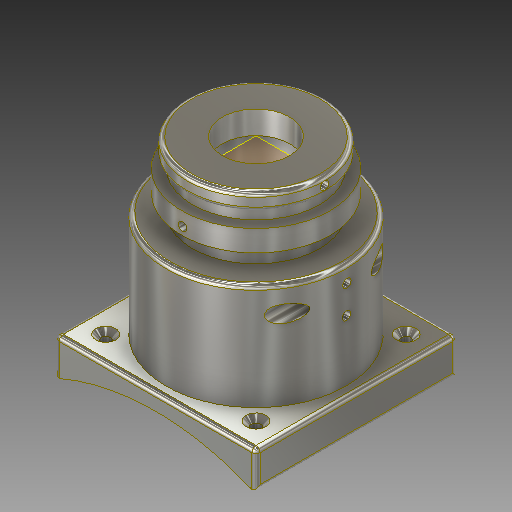
# Autodesk Inventor part: wyciag
Saved by Autodesk Inventor 2019.4 (Build 234330000, 330)
## iProperties
Created: 2019-06-01
Part Number: wyciag
Material: Silver
Document SubType Name: Modeling
Designer: Esterka
Density: 10.49 g/cm^3
Appearance: Silver
Author: Esterka
Autodesk Inventor part; units mm, degrees
ref_plane "XZ Plane" through (0, 0, 0) normal (0, 1, 0) x (-1, 0, 0)
sketch "Sketch1" plane through (0, 0, 0) normal (0, 0, 1) x (1, 0, 0)
  line L0 (0, 0) -> (95, 0)
  line L1 (0, 0) -> (0, -18)
  line L2 (95, -18) -> (95, 0)
  arc A0 (95, -18) -> (0, -18) centre (47.5, -122.7318) ccw
  dimension "d0" = 95
  dimension "d22" = 18
  dimension "d23" = 230
  dimension "d83" = 90
  dimension "d84" = 47.5
  constraints: 6 end point, 2 point on circle, 1 centre point, 1 horizontal, 1 vertical
  measures "d0" distance of L0.start L0.end
  measures "d22" distance of L0.start L1.end
  measures "d23" diameter of A0
  measures "d83" angle of L0 L2
  measures "d84" horizontal distance of L0.end A0.centre
extrude "Extrusion1" add sketch "Sketch1" along normal blind 95
fillet "Fillet1" radius 2 4 edges at (47.5, 0, 0) (0, 0, 47.5) (47.5, 0, 95) (95, 0, 47.5)
sketch "Sketch2" plane through (2, 0, 2) normal (0, 1, 0) x (1, 0, 0)
  line L0 (-1, 0) -> (-1, -98) projected
  circle A0 centre (45.5, -45.5) radius 42.5
  line L1 (93, 2) -> (-2, 2) projected
  line L2 (-2, 2) -> (-2, -93) projected
  dimension "d7" = 85
  dimension "d26" = 47.5
  dimension "d27" = 47.5
  constraints: 1 centre point, 1 coincident
  measures "d7" diameter of A0
  measures "d26" distance from line of L1 point (45.5, -45.5)
  measures "d27" distance from line of L2 point (45.5, -45.5)
extrude "Extrusion2" add sketch "Sketch2" along normal blind 50
sketch "Sketch3" plane through (47.5, 50, 47.5) normal (0, 1, 0) x (1, 0, 0)
  circle A0 centre (0, 0) radius 30
  point P0 (-47.5, 47.5)
  dimension "d10" = 60
  constraints: 1 centre point
  measures "d10" diameter of A0
extrude "Extrusion3" add sketch "Sketch3" along normal blind 23
fillet "Fillet2" radius 2 1 edges at (5, 50, 47.5)
ref_plane "Work Plane1" through (47.5, 68, 47.5) normal (0, 1, 0) x (1, 0, 0)
sketch "Sketch4" plane through (47.5, 68, 47.5) normal (0, 1, 0) x (1, 0, 0)
  circle A0 centre (0, 0) radius 35
  point P0 (-47.5, 47.5)
  dimension "d15" = 70
  constraints: 1 centre point
  measures "d15" diameter of A0
extrude "Extrusion4" add sketch "Sketch4" against normal blind 10
sketch "Sketch5" plane through (47.5, 73, 47.5) normal (0, 1, 0) x (1, 0, 0)
  circle A0 centre (0, 0) radius 32.5
  point P0 (-47.5, 47.5)
  dimension "d18" = 65
  constraints: 1 centre point
  measures "d18" diameter of A0
extrude "Extrusion5" add sketch "Sketch5" along normal blind 8
sketch "Sketch6" plane through (47.5, 81, 47.5) normal (0, 1, 0) x (1, 0, 0)
  circle A0 centre (0, 0) radius 15.875
  point P0 (-47.5, 47.5)
  dimension "d21" = 31.75
  constraints: 1 centre point
  measures "d21" diameter of A0
fillet "Fillet3" radius 2 10 edges at (95, -10, 95) (95, -18, 47.5) (95, -10, 0) (94.4142, -0.5858, 94.4142) (94.4142, -0.5858, 0.5858) (0, -10, 0) (0, -18, 47.5) (0, -10, 95) (0.5858, -0.5858, 0.5858) (0.5858, -0.5858, 94.4142)
fillet "Fillet4" radius 2 2 edges at (15, 73, 47.5) (15, 81, 47.5)
extrude "Extrusion6" cut sketch "Sketch6" against normal blind 128.575
sketch "Sketch7" plane through (0, 0, 0) normal (0, 0, 1) x (1, 0, 0)
  point P0 (0, 0)
  point P1 (83.4711, 37.711)
hole "Hole1" at (83.4711, 37.711, 0) direction (0, 0, 1) diameter 8 depth 146.3436 tip angle 118
sketch "Sketch8" plane through (0, 0, 0) normal (1, 0, 0) x (0, 1, 0)
  point P0 (0, 0)
  point P1 (62.0309, 49.7073)
hole "Hole2" at (0, 62.0309, 49.7073) direction (1, 0, 0) diameter 4 depth 30.4561 tip angle 118
sketch "Sketch9" plane through (0, 0, 0) normal (1, 0, 0) x (0, 1, 0)
  point P0 (0, 0)
ref_plane "Work Plane2" through (90, 0, 47.5) normal (1, 0, 0) x (0, 1, 0)
sketch "Sketch10" plane through (90, 0, 47.5) normal (1, 0, 0) x (0, 1, 0)
  point P0 (0, -47.5)
  point P1 (77.1141, 0)
hole "Hole3" at (90, 77.1141, 47.5) direction (-1, 0, 0) diameter 4 depth 30.4561 tip angle 118
ref_plane "Work Plane3" through (47.5, 0, 90) normal (0, 0, 1) x (1, 0, 0)
sketch "Sketch11" plane through (47.5, 0, 90) normal (0, 0, 1) x (1, 0, 0)
  point P0 (-47.5, 0)
  point P1 (0.3106, 61.752)
hole "Hole4" at (47.8106, 61.752, 90) direction (0, 0, -1) diameter 4 depth 30.4561 tip angle 118
sketch "Sketch12" plane through (90, 0, 47.5) normal (1, 0, 0) x (0, 1, 0)
  point P0 (0, -47.5)
  point P1 (41.8458, -0.5348)
  point P2 (28.7287, -0.2242)
hole "Hole5" at (90, 41.8458, 46.9652) at (90, 28.7287, 47.2758) direction (-1, 0, 0) diameter 4 depth 30.4561 tip angle 118
sketch "Sketch13" plane through (2, 0, 2) normal (0, 1, 0) x (1, 0, 0)
  line L0 (0, -93) -> (91, -93) projected
  line L1 (-2, 0) -> (-2, -91) projected
  line L2 (91, 2) -> (0, 2) projected
  line L3 (93, -91) -> (93, 0) projected
  point P0 (-2, 2)
  point P1 (10, -81)
  point P2 (10, -10)
  point P3 (81, -10)
  point P4 (81, -81)
  dimension "d65" = 12
  dimension "d66" = 12
  dimension "d67" = 12
  dimension "d68" = 12
  dimension "d69" = 12
  dimension "d70" = 12
  dimension "d71" = 12
  dimension "d72" = 12
  measures "d65" distance from line of L0 point (10, -81)
  measures "d66" distance from line of L1 point (10, -81)
  measures "d67" distance from line of L1 point (10, -10)
  measures "d68" distance from line of L2 point (10, -10)
  measures "d69" distance from line of L2 point (81, -10)
  measures "d70" distance from line of L3 point (81, -10)
  measures "d71" distance from line of L3 point (81, -81)
  measures "d72" distance from line of L0 point (81, -81)
hole "Hole6" at (83, 0, 83) at (83, 0, 12) at (12, 0, 83) at (12, 0, 12) direction (0, -1, 0) diameter 4.5 depth 30.4561 tip angle 118 countersink diameter 9.4 countersink angle 90 clearance for "Countersunk Flat Head Screw ISO 2009/7046" size "M4" standard "ISO"
sketch "Sketch14" plane through (0, 0, 0) normal (0, 1, 0) x (-1, 0, 0)
  circle A0 centre (-47.5, 47.5) radius 15.875 projected
  circle A1 centre (-47.5, 47.5) radius 25.4
  point P0 (0, 0)
  dimension "d80" = 50.8
  constraints: 1 centre point, 1 coincident
  measures "d80" diameter of A1
extrude "Extrusion7" cut sketch "Sketch14" along normal mid plane 140.175
body "Solid1"
